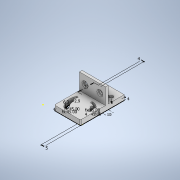
# Autodesk Inventor part: Printer_Mount
Saved by Autodesk Inventor 2022 (Build 260153000, 153)
## iProperties
Created: 2024-03-06
Part Number: Printer_Mount
Material: Generic
Document SubType Name: Modeling
Designer: Gotham City
Density: 1 g/cm^3
Appearance: Default
Author: Gotham City
Autodesk Inventor part; units mm, degrees
ref_plane "YZ Plane" through (0, 0, 0) normal (1, 0, 0) x (0, 1, 0)
ref_plane "XZ Plane" through (0, 0, 0) normal (0, 1, 0) x (-1, 0, 0)
ref_plane "XY Plane" through (0, 0, 0) normal (0, 0, 1) x (1, 0, 0)
sketch "Sketch5" plane through (0, 0, 0) normal (0, 1, 0) x (-1, 0, 0)
  line L0 (-17.367239, -42.08918) -> (-58.367239, -42.08918)
  circle A0 centre (-55.339239, -22.08918) radius 1.5
  line L1 (-58.367239, -42.08918) -> (-58.367239, -4.08918)
  circle A1 centre (-55.367239, -31.08918) radius 1.35
  circle A2 centre (-25.367239, -31.08918) radius 1.35
  line L2 (-58.367239, -4.08918) -> (-17.367239, -4.08918)
  line L3 (-17.367239, -4.08918) -> (-17.367239, -42.08918)
  circle A3 centre (-25.372239, -22.08918) radius 1.5
  line L4 (-25.367239, -31.08918) -> (-55.367239, -31.08918) construction
  line L5 (-25.372239, -22.08918) -> (-55.339239, -22.08918) construction
  point P0 (0, 0)
  dimension "d40" = 30
  dimension "d41" = 29.967
  dimension "d42" = 2.7
  dimension "d43" = 2.7
  dimension "d44" = 3
  dimension "d45" = 3
  dimension "d46" = 8
  dimension "d47" = 8.005
  dimension "d48" = 11
  dimension "d49" = 9
  dimension "d50" = 41
  dimension "d51" = 38
  constraints: 12 end point, 4 centre point
  measures "d40" distance of L4.end L4.start
  measures "d41" distance of L5.start L5.end
  measures "d42" diameter of A2
  measures "d43" diameter of A1
  measures "d44" diameter of A3
  measures "d45" diameter of A0
  measures "d46" distance from line of L3 L4.start
  measures "d47" distance from line of L3 L5.start
  measures "d48" distance from line of L4.start L0
  measures "d49" distance of L4.start L5.start
  measures "d50" distance of L0.end L0.start
  measures "d51" distance of L0.start L2.end
sketch "Sketch1" plane through (0, 0, 0) normal (0, 1, 0) x (-1, 0, 0)
  line L0 (-92.105786, -21.93918) -> (-104.16577, -21.93918) construction
  line L1 (-25.367239, -31.08918) -> (-55.367239, -31.08918) construction
  line L2 (-44.903739, -21.93918) -> (-44.903739, -31.08918) construction
  line L3 (-25.367239, -31.08918) -> (-55.367239, -31.08918) construction
  circle A0 centre (-25.367239, -31.08918) radius 1.35 construction
  circle A1 centre (-55.367239, -31.08918) radius 1.35 construction
  point P0 (0, 0)
  point P1 (-36.195239, -21.93918)
  point P2 (-53.612239, -21.93918)
  point P3 (-26.381239, -21.93918)
  dimension "d4" = 17.417
  dimension "d100" = 9.15
  dimension "d101" = 1.014
  dimension "d102" = 9.814
  constraints: 6 end point, 5 point on line, 2 horizontal, 1 collinear, 1 perpendicular, 1 symmetric about line
  measures "d4" distance of point (-53.612, -21.939) point (-36.195, -21.939)
  measures "d100" distance from line of point (-36.195, -21.939) L3
  measures "d101" horizontal distance of L1.start point (-26.381, -21.939)
  measures "d102" distance of point (-26.381, -21.939) point (-36.195, -21.939)
sketch "Sketch6" plane through (0, 0, 0) normal (0, 1, 0) x (-1, 0, 0)
  circle A0 centre (-25.372239, -22.08918) radius 3.15 construction
  circle A1 centre (-55.339239, -22.08918) radius 2 construction
  circle A2 centre (-25.367239, -31.08918) radius 1.45 construction
  circle A3 centre (-55.367239, -31.08918) radius 1.45 construction
  line L0 (-25.367239, -31.08918) -> (-44.903739, -21.93918) construction
  line L1 (-30.986817, -8.23439) -> (-44.903739, -21.93918) construction
  line L2 (-25.372239, -22.08918) -> (-44.903739, -21.93918) construction
  line L3 (-55.367239, -31.08918) -> (-44.903739, -21.93918) construction
  line L4 (-45.832524, -35.808019) -> (-44.903739, -21.93918) construction
  line L5 (-55.339239, -22.08918) -> (-44.903739, -21.93918) construction
  line L6 (-52.176686, -29.424259) -> (-44.903739, -21.93918) construction
  line L7 (-24.61932, -14.594816) -> (-44.903739, -21.93918) construction
  arc A4 (-55.367239, -31.08918) -> (-45.832524, -35.808019) centre (-44.903739, -21.93918) ccw construction
  arc A5 (-55.339239, -22.08918) -> (-52.176686, -29.424259) centre (-44.903739, -21.93918) ccw construction
  arc A6 (-25.372239, -22.08918) -> (-30.986817, -8.23439) centre (-44.903739, -21.93918) ccw construction
  arc A7 (-25.367239, -31.08918) -> (-24.61932, -14.594816) centre (-44.903739, -21.93918) ccw construction
  point P0 (0, 0)
  dimension "d56" = 2.9
  dimension "d57" = 2.9
  dimension "d58" = 6.3
  dimension "d59" = 4
  dimension "d110" = 45
  dimension "d111" = 45
  dimension "d112" = 45
  dimension "d113" = 45
  constraints: 17 end point, 9 coincident, 8 centre point, 8 point on circle, 3 other
  measures "d56" diameter of A2
  measures "d57" diameter of A3
  measures "d58" diameter of A0
  measures "d59" diameter of A1
  measures "d110" angle of L6 L5
  measures "d111" angle of L4 L3
  measures "d112" angle of L7 L0
  measures "d113" angle of L1 L2
sketch "Sketch3" plane through (0, 0, 0) normal (0, 1, 0) x (-1, 0, 0)
  arc A0 (-55.339239, -22.08918) -> (-52.176686, -29.424259) centre (-44.903739, -21.93918) ccw construction
  arc A1 (-55.367239, -31.08918) -> (-45.832524, -35.808019) centre (-44.903739, -21.93918) ccw construction
  arc A2 (-25.367239, -31.08918) -> (-24.61932, -14.594816) centre (-44.903739, -21.93918) ccw construction
  arc A3 (-25.372239, -22.08918) -> (-30.986817, -8.23439) centre (-44.903739, -21.93918) ccw construction
  arc A4 (-22.222332, -22.113371) -> (-28.742391, -6.024175) centre (-44.903739, -21.93918) ccw
  arc A5 (-28.522146, -22.064989) -> (-33.231243, -10.444605) centre (-44.903739, -21.93918) ccw
  arc A6 (-24.054124, -31.704183) -> (-23.255935, -14.101176) centre (-44.903739, -21.93918) ccw
  arc A7 (-26.680354, -30.474177) -> (-25.982706, -15.088455) centre (-44.903739, -21.93918) ccw
  arc A8 (-53.339446, -22.060435) -> (-50.782944, -27.989866) centre (-44.903739, -21.93918) ccw
  arc A9 (-57.339032, -22.117925) -> (-53.570427, -30.858652) centre (-44.903739, -21.93918) ccw
  arc A10 (-54.275715, -30.134677) -> (-45.735635, -34.36126) centre (-44.903739, -21.93918) ccw
  arc A11 (-56.458763, -32.043683) -> (-45.929412, -37.254778) centre (-44.903739, -21.93918) ccw
  arc A12 (-53.339446, -22.060435) -> (-57.339032, -22.117925) centre (-55.339239, -22.08918) ccw
  arc A13 (-53.570427, -30.858652) -> (-50.782944, -27.989866) centre (-52.176686, -29.424259) ccw
  arc A14 (-45.929412, -37.254778) -> (-45.735635, -34.36126) centre (-45.832524, -35.808019) ccw
  arc A15 (-54.275715, -30.134677) -> (-56.458763, -32.043683) centre (-55.367239, -31.08918) ccw
  arc A16 (-26.680354, -30.474177) -> (-24.054124, -31.704183) centre (-25.367239, -31.08918) ccw
  arc A17 (-23.255935, -14.101176) -> (-25.982706, -15.088455) centre (-24.61932, -14.594816) ccw
  arc A18 (-28.522146, -22.064989) -> (-22.222332, -22.113371) centre (-25.372239, -22.08918) ccw
  arc A19 (-28.742391, -6.024175) -> (-33.231243, -10.444605) centre (-30.986817, -8.23439) ccw
  circle A20 centre (-25.372239, -22.08918) radius 3.15 construction
  circle A21 centre (-25.367239, -31.08918) radius 1.45 construction
  circle A22 centre (-55.339239, -22.08918) radius 2 construction
  circle A23 centre (-55.367239, -31.08918) radius 1.45 construction
  point P0 (-25.050364, -25.222692)
  point P1 (-23.921592, -13.323723)
  constraints: 33 point on circle, 16 centre point, 16 tangent, 8 coincident, 8 other
sketch "Sketch2" plane through (0, 0, 0) normal (0, 1, 0) x (-1, 0, 0)
  line L0 (-17.880669, -1.08439) -> (-61.339239, -1.08439)
  line L1 (-61.339239, -1.08439) -> (-61.339239, -74.258019)
  line L2 (-61.339239, -74.258019) -> (-17.880669, -74.258019)
  line L3 (-17.880669, -74.258019) -> (-17.880669, -1.08439)
  circle A0 centre (-53.839239, -60.758019) radius 2.5 construction
  line L4 (-56.339239, -1.08439) -> (-56.339239, -74.258019) construction
  line L5 (-39.609954, -1.08439) -> (-39.609954, -74.258019) construction
  line L6 (-61.339239, -58.258019) -> (-39.609954, -58.258019) construction
  line L7 (-39.609954, -58.258019) -> (-17.880669, -58.258019) construction
  circle A1 centre (-25.380669, -60.758019) radius 2.5 construction
  line L8 (-61.339239, -63.258019) -> (-17.880669, -63.258019) construction
  line L9 (-61.339239, -37.258019) -> (-17.880669, -37.258019) construction
  line L10 (-61.339239, -47.258019) -> (-17.880669, -47.258019) construction
  circle A2 centre (-55.339239, -22.08918) radius 2 construction
  line L11 (-57.339239, -1.08439) -> (-57.339239, -74.258019) construction
  line L12 (-21.880669, -74.258019) -> (-21.880669, -1.08439) construction
  line L13 (-17.880669, -5.08439) -> (-61.339239, -5.08439) construction
  line L14 (-53.839239, -60.758019) -> (-53.839239, -74.258019) construction
  line L15 (-53.839239, -60.758019) -> (-53.839239, -47.258019) construction
  arc A3 (-45.929412, -37.254778) -> (-45.735635, -34.36126) centre (-45.832524, -35.808019) ccw construction
  arc A4 (-28.742391, -6.024175) -> (-33.231243, -10.444605) centre (-30.986817, -8.23439) ccw construction
  arc A5 (-24.054124, -31.704183) -> (-23.255935, -14.101176) centre (-44.903739, -21.93918) ccw construction
  point P0 (-58.367239, -4.08918)
  dimension "d25" = 5
  dimension "d30" = 10
  dimension "d32" = 5
  dimension "d64" = 4
  dimension "d66" = 4
  dimension "d105" = 27
  dimension "d106" = 4
  constraints: 32 end point, 19 point on line, 13 perpendicular, 7 tangent, 2 centre point, 2 collinear, 2 midpoint, 2 parallel, 1 horizontal, 1 symmetric about line, 1 other
  measures "d25" diameter of A0
  measures "d30" distance between parallel lines of L9 L10
  measures "d32" distance between parallel lines of L1 L4
  measures "d64" distance between parallel lines of L3 L12
  measures "d66" distance between parallel lines of L1 L11
  measures "d105" distance between parallel lines of L2 L10
  measures "d106" distance between parallel lines of L13 L0
extrude "Extrusion1" add sketch "Sketch2" along normal blind 8
extrude "Extrusion2" cut sketch "Sketch3" along normal through all
hole "Hole1" at (53.839239, 0, -60.758019) at (25.380669, 0, -60.758019) direction (0, 1, 0) diameter 5.5 end through all
fillet "Fillet1" radius 2 2 edges at (61.3392, 4, -1.0844) (17.8807, 4, -1.0844)
sketch "Sketch8" plane through (0, 0, 0) normal (0, -1, 0) x (1, 0, 0)
  point P0 (0, 0)
sketch "Sketch7" plane through (0, 8, 0) normal (0, 1, 0) x (-1, 0, 0)
  line L0 (-17.880669, -27.23918) -> (-61.339239, -27.23918)
  line L1 (-61.339239, -27.23918) -> (-61.339239, -34.93918)
  line L2 (-61.339239, -34.93918) -> (-17.880669, -34.93918)
  line L3 (-17.880669, -34.93918) -> (-17.880669, -27.23918)
  circle A0 centre (-25.372239, -22.08918) radius 3.15 construction
  circle A1 centre (-53.839239, -60.758019) radius 2.75 construction
  circle A2 centre (-25.380669, -60.758019) radius 2.75 construction
  line L4 (-61.339239, -74.258019) -> (-17.880669, -74.258019) construction
  line L5 (-17.880669, -74.258019) -> (-17.880669, -3.08439) construction
  line L6 (-19.880669, -1.08439) -> (-59.339239, -1.08439) construction
  line L7 (-61.339239, -3.08439) -> (-61.339239, -74.258019) construction
  line L8 (-25.367239, -31.08918) -> (-55.367239, -31.08918) construction
  circle A3 centre (-55.367239, -31.08918) radius 1.35 construction
  circle A4 centre (-25.367239, -31.08918) radius 1.35 construction
  line L9 (-17.880669, -74.258019) -> (-17.880669, -3.08439) construction
  line L10 (-61.339239, -3.08439) -> (-61.339239, -74.258019) construction
  arc A5 (-17.880669, -3.08439) -> (-19.880669, -1.08439) centre (-19.880669, -3.08439) ccw
  arc A6 (-59.339239, -1.08439) -> (-61.339239, -3.08439) centre (-59.339239, -3.08439) ccw
  point P0 (0, 0)
  point P1 (-64.253643, -73.673599)
  point P2 (-18.221663, -73.673599)
  point P3 (-17.880669, -1.08439)
  point P4 (-61.339239, -1.08439)
  dimension "d68" = 5.15
  constraints: 8 end point, 2 parallel, 1 horizontal, 1 perpendicular, 5 other
  measures "d68" distance from line of L0 A0.centre
extrude "Extrusion3" add sketch "Sketch7" along normal blind 2 separate body
sketch "Sketch9" plane through (0, 8, 0) normal (0, -1, 0) x (1, 0, 0)
  line L0 (17.880669, -74.258019) -> (17.880669, -3.08439) construction
  line L1 (61.339239, -3.08439) -> (61.339239, -74.258019)
  line L2 (17.880669, -42.894505) -> (61.339239, -42.894505)
  line L3 (61.339239, -42.894505) -> (61.339239, -47.258019)
  line L4 (61.339239, -47.258019) -> (17.880669, -47.258019)
  line L5 (17.880669, -47.258019) -> (17.880669, -47.258019)
  line L6 (61.339239, -47.258019) -> (17.880669, -47.258019) construction
  line L7 (61.339239, -37.258019) -> (17.880669, -37.258019) construction
  line L8 (17.880669, -42.894505) -> (17.880669, -47.258019)
  line L9 (61.339239, -34.93918) -> (17.880669, -34.93918) construction
  line L10 (44.903739, -21.93918) -> (61.339239, -34.93918) construction
  line L11 (44.903739, -21.93918) -> (47.333004, -42.753222) construction
  arc A0 (47.333004, -42.753222) -> (61.339239, -34.93918) centre (44.903739, -21.93918) ccw construction
  point P0 (0, 0)
  point P1 (17.880669, -1.08439)
  point P2 (61.339239, -1.08439)
  point P3 (61.339239, -42.894505)
  point P4 (17.880669, -27.23918)
  dimension "d114" = 45
  constraints: 14 end point, 2 parallel, 2 point on circle, 2 point on line, 1 centre point, 1 coincident, 1 horizontal, 1 perpendicular, 1 tangent, 1 vertical
  measures "d114" angle of L10 L11
extrude "Extrusion4" add sketch "Sketch9" against normal blind 27
fillet "Fillet2" radius 2 4 edges at (17.8807, 9, -34.9392) (17.8807, 9, -27.2392) (61.3392, 9, -27.2392) (61.3392, 9, -34.9392)
sketch "Sketch10" plane through (0, 10, 0) normal (0, 1, 0) x (1, 0, 0)
  circle A0 centre (55.367239, 31.08918) radius 1.35
  circle A1 centre (25.367239, 31.08918) radius 1.35
  point P0 (0, 0)
extrude "Extrusion5" cut sketch "Sketch10" against normal through all
sketch "Sketch11" plane through (18.310269, 0, -42.894505) normal (0, 0, 1) x (-1, 0, 0)
  circle A0 centre (-8.799685, -21.5) radius 2.5 construction
  line L0 (0.429599, -21.5) -> (-43.02897, -21.5) construction
  circle A1 centre (-33.799685, -21.5) radius 2.5 construction
  line L1 (0.429599, -35) -> (-43.02897, -35) construction
  line L2 (-21.299685, -21.5) -> (-21.299685, -8) construction
  line L3 (-21.299685, -21.5) -> (-21.299685, -35) construction
  line L4 (0.429599, -8) -> (0.429599, -35) construction
  line L5 (-43.02897, -8) -> (-43.02897, -35) construction
  point P0 (18.310269, 0)
  dimension "d81" = 5
  dimension "d83" = 25
  constraints: 6 end point, 4 midpoint, 2 centre point, 2 point on line, 1 collinear, 1 equal radius, 1 horizontal, 1 symmetric about line, 1 vertical
  measures "d81" diameter of A0
  measures "d83" distance of A1.centre A0.centre
hole "Hole2" at (52.109954, 21.5, -42.894505) at (27.109954, 21.5, -42.894505) direction (0, 0, -1) diameter 5.5 end through all counterbore diameter 10 counterbore depth 2 clearance for "Socket Head Cap Screw ISO 4762" size "M5" standard "ISO"
thicken "Thicken1" operation add thickness 0.07 both sides no extend neighbours yes toward (-0.9532105, 0, -0.3023073) faces at (22.957906, 5.333333, -28.899221) (23.352214, 5.333333, -13.889875) (24.741692, 5.333333, -11.548394) (29.125999, 5.333333, -5.692765) (29.047774, 5.333333, -17.820834) (28.485729, 5.333333, -22.567384) (25.778207, 5.333333, -28.196333) (26.786458, 5.333333, -31.386364)
thicken "Thicken2" operation add thickness 0.07 both sides no extend neighbours yes toward (0.126258, 0, -0.9919974) faces at (52.429202, 5.333333, -31.408254) (52.148648, 5.333333, -26.262043) (55.923227, 5.333333, -20.17634) (55.583646, 5.333333, -28.311625)
thicken "Thicken3" operation add thickness 0.07 both sides no extend neighbours yes toward (-0.2123404, 0, 0.9771958) faces at (47.547357, 2.666667, -34.105173) (44.415929, 5.333333, -35.498568) (55.773156, 2.666667, -32.777783) (56.102548, 5.333333, -29.839452)
body "Solid1"
body "Solid2"
